Autodesk Inventor part; units mm, degrees
(part 2 of 2)
  line L983 (37.6555, 15.8013) -> (37.6555, 16.1823)
  line L984 (36.3398, 14.9098) -> (36.7208, 14.9098)
  line L985 (36.5303, 14.7193) -> (36.5303, 15.1003)
  line L986 (36.3398, 15.9918) -> (36.7208, 15.9918)
  line L987 (36.5303, 15.8013) -> (36.5303, 16.1823)
  line L988 (35.2146, 14.9098) -> (35.5956, 14.9098)
  line L989 (35.4051, 14.7193) -> (35.4051, 15.1003)
  line L990 (35.2146, 15.9918) -> (35.5956, 15.9918)
  line L991 (35.4051, 15.8013) -> (35.4051, 16.1823)
  line L992 (34.0893, 17.0713) -> (34.4703, 17.0713)
  line L993 (34.2798, 16.8808) -> (34.2798, 17.2618)
  line L994 (36.3398, 17.0713) -> (36.7208, 17.0713)
  line L995 (36.5303, 16.8808) -> (36.5303, 17.2618)
  line L996 (34.0893, 15.9918) -> (34.4703, 15.9918)
  line L997 (34.2798, 15.8013) -> (34.2798, 16.1823)
  line L998 (35.2146, 17.0713) -> (35.5956, 17.0713)
  line L999 (35.4051, 16.8808) -> (35.4051, 17.2618)
  line L1000 (37.465, 17.0713) -> (37.846, 17.0713)
  line L1001 (37.6555, 16.8808) -> (37.6555, 17.2618)
  line L1002 (38.5902, 17.0713) -> (38.9712, 17.0713)
  line L1003 (38.7807, 16.8808) -> (38.7807, 17.2618)
  line L1004 (34.0893, 14.9098) -> (34.4703, 14.9098)
  line L1005 (34.2798, 14.7193) -> (34.2798, 15.1003)
  line L1006 (34.0893, 13.7617) -> (34.4703, 13.7617)
  line L1007 (34.2798, 13.5712) -> (34.2798, 13.9522)
  line L1008 (38.5902, 11.6002) -> (38.9712, 11.6002)
  line L1009 (38.7807, 11.4097) -> (38.7807, 11.7907)
  line L1010 (37.465, 11.6002) -> (37.846, 11.6002)
  line L1011 (37.6555, 11.4097) -> (37.6555, 11.7907)
  line L1012 (35.2146, 11.6002) -> (35.5956, 11.6002)
  line L1013 (35.4051, 11.4097) -> (35.4051, 11.7907)
  line L1014 (34.0893, 12.6822) -> (34.4703, 12.6822)
  line L1015 (34.2798, 12.4917) -> (34.2798, 12.8727)
  line L1016 (36.3398, 11.6002) -> (36.7208, 11.6002)
  line L1017 (36.5303, 11.4097) -> (36.5303, 11.7907)
  line L1018 (34.0893, 11.6002) -> (34.4703, 11.6002)
  line L1019 (34.2798, 11.4097) -> (34.2798, 11.7907)
  line L1020 (35.2146, 12.6822) -> (35.5956, 12.6822)
  line L1021 (35.4051, 12.4917) -> (35.4051, 12.8727)
  line L1022 (35.2146, 13.7617) -> (35.5956, 13.7617)
  line L1023 (35.4051, 13.5712) -> (35.4051, 13.9522)
  line L1024 (36.3398, 12.6822) -> (36.7208, 12.6822)
  line L1025 (36.5303, 12.4917) -> (36.5303, 12.8727)
  line L1026 (36.3398, 13.7617) -> (36.7208, 13.7617)
  line L1027 (36.5303, 13.5712) -> (36.5303, 13.9522)
  line L1028 (37.465, 12.6822) -> (37.846, 12.6822)
  line L1029 (37.6555, 12.4917) -> (37.6555, 12.8727)
  line L1030 (37.465, 13.7617) -> (37.846, 13.7617)
  line L1031 (37.6555, 13.5712) -> (37.6555, 13.9522)
  line L1032 (38.5902, 12.6822) -> (38.9712, 12.6822)
  line L1033 (38.7807, 12.4917) -> (38.7807, 12.8727)
  line L1034 (38.5902, 13.7617) -> (38.9712, 13.7617)
  line L1035 (38.7807, 13.5712) -> (38.7807, 13.9522)
  line L1036 (38.5902, 10.5207) -> (38.9712, 10.5207)
  line L1037 (38.7807, 10.3302) -> (38.7807, 10.7112)
  line L1038 (37.465, 10.5207) -> (37.846, 10.5207)
  line L1039 (37.6555, 10.3302) -> (37.6555, 10.7112)
  line L1040 (36.3398, 10.5207) -> (36.7208, 10.5207)
  line L1041 (36.5303, 10.3302) -> (36.5303, 10.7112)
  line L1042 (35.2146, 10.5207) -> (35.5956, 10.5207)
  line L1043 (35.4051, 10.3302) -> (35.4051, 10.7112)
  line L1044 (34.0893, 9.4412) -> (34.4703, 9.4412)
  line L1045 (34.2798, 9.2507) -> (34.2798, 9.6317)
  line L1046 (36.3398, 9.4412) -> (36.7208, 9.4412)
  line L1047 (36.5303, 9.2507) -> (36.5303, 9.6317)
  line L1048 (34.0893, 10.5207) -> (34.4703, 10.5207)
  line L1049 (34.2798, 10.3302) -> (34.2798, 10.7112)
  line L1050 (35.2146, 9.4412) -> (35.5956, 9.4412)
  line L1051 (35.4051, 9.2507) -> (35.4051, 9.6317)
  line L1052 (37.465, 9.4412) -> (37.846, 9.4412)
  line L1053 (37.6555, 9.2507) -> (37.6555, 9.6317)
  line L1054 (38.5902, 9.4412) -> (38.9712, 9.4412)
  line L1055 (38.7807, 9.2507) -> (38.7807, 9.6317)
  line L1056 (38.5902, 19.2303) -> (38.9712, 19.2303)
  line L1057 (38.7807, 19.0398) -> (38.7807, 19.4208)
  line L1058 (37.465, 19.2303) -> (37.846, 19.2303)
  line L1059 (37.6555, 19.0398) -> (37.6555, 19.4208)
  line L1060 (35.2146, 19.2303) -> (35.5956, 19.2303)
  line L1061 (35.4051, 19.0398) -> (35.4051, 19.4208)
  line L1062 (34.0893, 18.1508) -> (34.4703, 18.1508)
  line L1063 (34.2798, 17.9603) -> (34.2798, 18.3413)
  line L1064 (36.3398, 19.2303) -> (36.7208, 19.2303)
  line L1065 (36.5303, 19.0398) -> (36.5303, 19.4208)
  line L1066 (34.0893, 19.2303) -> (34.4703, 19.2303)
  line L1067 (34.2798, 19.0398) -> (34.2798, 19.4208)
  line L1068 (35.2146, 18.1508) -> (35.5956, 18.1508)
  line L1069 (35.4051, 17.9603) -> (35.4051, 18.3413)
  line L1070 (36.3398, 18.1508) -> (36.7208, 18.1508)
  line L1071 (36.5303, 17.9603) -> (36.5303, 18.3413)
  line L1072 (37.465, 18.1508) -> (37.846, 18.1508)
  line L1073 (37.6555, 17.9603) -> (37.6555, 18.3413)
  line L1074 (38.5902, 18.1508) -> (38.9712, 18.1508)
  line L1075 (38.7807, 17.9603) -> (38.7807, 18.3413)
  line L1076 (24.1935, 38.735) -> (24.5745, 38.735)
  line L1077 (24.384, 38.5445) -> (24.384, 38.9255)
  line L1078 (21.3995, 35.56) -> (21.7805, 35.56)
  line L1079 (21.59, 35.3695) -> (21.59, 35.7505)
  line L1080 (3.8735, 27.94) -> (4.2545, 27.94)
  line L1081 (4.064, 27.7495) -> (4.064, 28.1305)
  line L1082 (3.8735, 17.653) -> (4.2545, 17.653)
  line L1083 (4.064, 17.4625) -> (4.064, 17.8435)
  line L1084 (3.1115, 20.574) -> (3.4925, 20.574)
  line L1085 (3.302, 20.3835) -> (3.302, 20.7645)
  line L1086 (4.8895, 27.94) -> (5.2705, 27.94)
  line L1087 (5.08, 27.7495) -> (5.08, 28.1305)
  line L1088 (4.6355, 18.415) -> (5.0165, 18.415)
  line L1089 (4.826, 18.2245) -> (4.826, 18.6055)
  line L1090 (3.8735, 10.541) -> (4.2545, 10.541)
  line L1091 (4.064, 10.3505) -> (4.064, 10.7315)
  line L1092 (10.6045, 34.29) -> (10.9855, 34.29)
  line L1093 (10.795, 34.0995) -> (10.795, 34.4805)
  line L1094 (9.4615, 8.128) -> (9.8425, 8.128)
  line L1095 (9.652, 7.9375) -> (9.652, 8.3185)
  line L1096 (7.8105, 13.081) -> (8.1915, 13.081)
  line L1097 (8.001, 12.8905) -> (8.001, 13.2715)
  line L1098 (47.8155, 27.94) -> (48.1965, 27.94)
  line L1099 (48.006, 27.7495) -> (48.006, 28.1305)
  line L1100 (12.446, 26.4414) -> (12.954, 26.4414)
  line L1101 (12.7, 26.1874) -> (12.7, 26.6954)
  line L1102 (19.2405, 47.5107) -> (19.6215, 47.5107)
  line L1103 (19.431, 47.3202) -> (19.431, 47.7012)
  line L1104 (18.7325, 11.303) -> (19.1135, 11.303)
  line L1105 (18.923, 11.1125) -> (18.923, 11.4935)
  line L1106 (18.2245, 10.414) -> (18.6055, 10.414)
  line L1107 (18.415, 10.2235) -> (18.415, 10.6045)
  line L1108 (18.2245, 9.398) -> (18.6055, 9.398)
  line L1109 (18.415, 9.2075) -> (18.415, 9.5885)
  line L1110 (23.5585, 11.176) -> (23.9395, 11.176)
  line L1111 (23.749, 10.9855) -> (23.749, 11.3665)
  line L1112 (18.0975, 6.223) -> (18.4785, 6.223)
  line L1113 (18.288, 6.0325) -> (18.288, 6.4135)
  line L1114 (16.7005, 50.038) -> (17.0815, 50.038)
  line L1115 (16.891, 49.8475) -> (16.891, 50.2285)
  line L1116 (9.7155, 43.053) -> (10.0965, 43.053)
  line L1117 (9.906, 42.8625) -> (9.906, 43.2435)
  line L1118 (12.5095, 43.053) -> (12.8905, 43.053)
  line L1119 (12.7, 42.8625) -> (12.7, 43.2435)
  line L1120 (5.3975, 26.035) -> (5.7785, 26.035)
  line L1121 (5.588, 25.8445) -> (5.588, 26.2255)
  line L1122 (6.1595, 25.4) -> (6.5405, 25.4)
  line L1123 (6.35, 25.2095) -> (6.35, 25.5905)
  line L1124 (7.8105, 25.4) -> (8.1915, 25.4)
  line L1125 (8.001, 25.2095) -> (8.001, 25.5905)
  line L1126 (7.0485, 24.638) -> (7.4295, 24.638)
  line L1127 (7.239, 24.4475) -> (7.239, 24.8285)
  line L1128 (8.5725, 26.035) -> (8.9535, 26.035)
  line L1129 (8.763, 25.8445) -> (8.763, 26.2255)
  line L1130 (28.7655, 14.3358) -> (29.1465, 14.3358)
  line L1131 (28.956, 14.1453) -> (28.956, 14.5263)
  line L1132 (28.4226, -3.4544) -> (27.4091, -3.4544)
  line L1133 (27.4091, -3.4544) -> (28.4226, -2.4384)
  line L1134 (28.4226, -2.4384) -> (28.4226, -2.1844)
  line L1135 (28.4226, -2.1844) -> (28.1711, -1.9304)
  line L1136 (28.1711, -1.9304) -> (27.6631, -1.9304)
  line L1137 (27.6631, -1.9304) -> (27.4091, -2.1844)
  line L1138 (29.9466, -1.9304) -> (28.9306, -1.9304)
  line L1139 (28.9306, -1.9304) -> (28.9306, -2.6924)
  line L1140 (28.9306, -2.6924) -> (29.4386, -2.4384)
  line L1141 (29.4386, -2.4384) -> (29.6926, -2.4384)
  line L1142 (29.6926, -2.4384) -> (29.9466, -2.6924)
  line L1143 (29.9466, -2.6924) -> (29.9466, -3.2004)
  line L1144 (29.9466, -3.2004) -> (29.6926, -3.4544)
  line L1145 (29.6926, -3.4544) -> (29.1846, -3.4544)
  line L1146 (29.1846, -3.4544) -> (28.9306, -3.2004)
  line L1147 (31.4706, -1.9304) -> (30.9626, -2.1844)
  line L1148 (30.9626, -2.1844) -> (30.4546, -2.6924)
  line L1149 (30.4546, -2.6924) -> (30.4546, -3.2004)
  line L1150 (30.4546, -3.2004) -> (30.7086, -3.4544)
  line L1151 (30.7086, -3.4544) -> (31.2166, -3.4544)
  line L1152 (31.2166, -3.4544) -> (31.4706, -3.2004)
  line L1153 (31.4706, -3.2004) -> (31.4706, -2.9464)
  line L1154 (31.4706, -2.9464) -> (31.2166, -2.6924)
  line L1155 (31.2166, -2.6924) -> (30.4546, -2.6924)
  line L1156 (31.9786, -2.1844) -> (32.2326, -1.9304)
  line L1157 (32.2326, -1.9304) -> (32.7406, -1.9304)
  line L1158 (32.7406, -1.9304) -> (32.9946, -2.1844)
  line L1159 (32.9946, -2.1844) -> (32.9946, -3.2004)
  line L1160 (32.9946, -3.2004) -> (32.7406, -3.4544)
  line L1161 (32.7406, -3.4544) -> (32.2326, -3.4544)
  line L1162 (32.2326, -3.4544) -> (31.9786, -3.2004)
  line L1163 (31.9786, -3.2004) -> (31.9786, -2.1844)
  line L1164 (33.5026, -3.4544) -> (33.5026, -2.4384)
  line L1165 (33.5026, -2.4384) -> (33.7566, -2.4384)
  line L1166 (33.7566, -2.4384) -> (34.0106, -2.6924)
  line L1167 (34.0106, -2.6924) -> (34.0106, -3.4544)
  line L1168 (34.0106, -3.4544) -> (34.0106, -2.6924)
  line L1169 (34.0106, -2.6924) -> (34.2646, -2.4384)
  line L1170 (34.2646, -2.4384) -> (34.5186, -2.6924)
  line L1171 (34.5186, -2.6924) -> (34.5186, -3.4544)
  line L1172 (35.0266, -3.4544) -> (35.5346, -3.4544)
  line L1173 (35.5346, -3.4544) -> (35.2806, -3.4544)
  line L1174 (35.2806, -3.4544) -> (35.2806, -2.4384)
  line L1175 (35.2806, -2.4384) -> (35.0266, -2.4384)
  line L1176 (36.2941, -3.4544) -> (36.8021, -3.4544)
  line L1177 (36.8021, -3.4544) -> (36.5481, -3.4544)
  line L1178 (36.5481, -3.4544) -> (36.5481, -1.9304)
  line L1179 (36.5481, -1.9304) -> (36.2941, -1.9304)
  line L1180 (-1.6256, 21.5646) -> (-1.6256, 20.5511)
  line L1181 (-1.6256, 20.5511) -> (-2.6416, 21.5646)
  line L1182 (-2.6416, 21.5646) -> (-2.8956, 21.5646)
  line L1183 (-2.8956, 21.5646) -> (-3.1496, 21.3106)
  line L1184 (-3.1496, 21.3106) -> (-3.1496, 20.8051)
  line L1185 (-3.1496, 20.8051) -> (-2.8956, 20.5511)
  line L1186 (-2.8956, 22.0726) -> (-3.1496, 22.3266)
  line L1187 (-3.1496, 22.3266) -> (-3.1496, 22.8346)
  line L1188 (-3.1496, 22.8346) -> (-2.8956, 23.0886)
  line L1189 (-2.8956, 23.0886) -> (-1.8796, 23.0886)
  line L1190 (-1.8796, 23.0886) -> (-1.6256, 22.8346)
  line L1191 (-1.6256, 22.8346) -> (-1.6256, 22.3266)
  line L1192 (-1.6256, 22.3266) -> (-1.8796, 22.0726)
  line L1193 (-1.8796, 22.0726) -> (-2.8956, 22.0726)
  line L1194 (-1.6256, 24.6126) -> (-1.6256, 23.5966)
  line L1195 (-1.6256, 23.5966) -> (-2.6416, 24.6126)
  line L1196 (-2.6416, 24.6126) -> (-2.8956, 24.6126)
  line L1197 (-2.8956, 24.6126) -> (-3.1496, 24.3586)
  line L1198 (-3.1496, 24.3586) -> (-3.1496, 23.8506)
  line L1199 (-3.1496, 23.8506) -> (-2.8956, 23.5966)
  line L1200 (-2.8956, 25.1206) -> (-3.1496, 25.3746)
  line L1201 (-3.1496, 25.3746) -> (-3.1496, 25.8826)
  line L1202 (-3.1496, 25.8826) -> (-2.8956, 26.1366)
  line L1203 (-2.8956, 26.1366) -> (-1.8796, 26.1366)
  line L1204 (-1.8796, 26.1366) -> (-1.6256, 25.8826)
  line L1205 (-1.6256, 25.8826) -> (-1.6256, 25.3746)
  line L1206 (-1.6256, 25.3746) -> (-1.8796, 25.1206)
  line L1207 (-1.8796, 25.1206) -> (-2.8956, 25.1206)
  line L1208 (-1.6256, 26.6446) -> (-2.6416, 26.6446)
  line L1209 (-2.6416, 26.6446) -> (-2.6416, 26.8986)
  line L1210 (-2.6416, 26.8986) -> (-2.3876, 27.1526)
  line L1211 (-2.3876, 27.1526) -> (-1.6256, 27.1526)
  line L1212 (-1.6256, 27.1526) -> (-2.3876, 27.1526)
  line L1213 (-2.3876, 27.1526) -> (-2.6416, 27.4066)
  line L1214 (-2.6416, 27.4066) -> (-2.3876, 27.6606)
  line L1215 (-2.3876, 27.6606) -> (-1.6256, 27.6606)
  line L1216 (-1.6256, 28.1686) -> (-1.6256, 28.6766)
  line L1217 (-1.6256, 28.6766) -> (-1.6256, 28.4226)
  line L1218 (-1.6256, 28.4226) -> (-2.6416, 28.4226)
  line L1219 (-2.6416, 28.4226) -> (-2.6416, 28.1686)
  line L1220 (-1.6256, 29.4361) -> (-1.6256, 29.9441)
  line L1221 (-1.6256, 29.9441) -> (-1.6256, 29.6901)
  line L1222 (-1.6256, 29.6901) -> (-3.1496, 29.6901)
  line L1223 (-3.1496, 29.6901) -> (-3.1496, 29.4361)
  line L1224 (0, 51.308) -> (65.024, 51.308)
  line L1225 (65.024, 51.308) -> (65.024, 0)
  line L1226 (65.024, 0) -> (0, 0)
  line L1227 (0, 0) -> (0, 51.308)
  circle A0 centre (3.81, 47.244) radius 1.6
  circle A1 centre (11.43, 4.064) radius 1.6
  dimension "d0" = 65.024
  dimension "d1" = 3.2
  dimension "d2" = 3.2
  constraints: 2456 end point, 2 centre point, 2 midpoint, 2 parallel, 1 horizontal, 1 perpendicular
  measures "d0" distance between parallel lines of L18 L16
  measures "d1" diameter of A0
  measures "d2" diameter of A1
extrude "押し出し1" add sketch "スケッチ1" along normal blind 1.2 contours L16 L17 L18 L19
